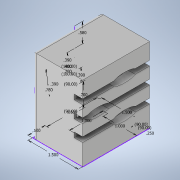
# Autodesk Inventor part: Valve Holder-3valve
Saved by Autodesk Inventor 2020 (Build 240168000, 168)
## iProperties
Created: 2022-01-25
Part Number: Valve Holder-3valve
Material: Generic
Document SubType Name: Modeling
Designer: Beaucage
Density: 1 g/cm^3
Appearance: Default
Author: Beaucage
Autodesk Inventor part; units mm, degrees
ref_plane "YZ Plane" through (0, 0, 0) normal (1, 0, 0) x (0, 1, 0)
ref_plane "XZ Plane" through (0, 0, 0) normal (0, 1, 0) x (-1, 0, 0)
ref_plane "XY Plane" through (0, 0, 0) normal (0, 0, 1) x (1, 0, 0)
sketch "Sketch1" plane through (0, 0, 0) normal (0, 1, 0) x (-1, 0, 0)
  line L0 (0, 0) -> (38.1, 0)
  line L1 (38.1, 0) -> (38.1, -38.1)
  line L2 (38.1, -38.1) -> (0, -38.1)
  line L3 (0, -38.1) -> (0, 0)
  line L4 (0, -38.1) -> (0, -31.75)
  line L5 (0, -38.1) -> (6.35, -38.1) construction
  line L6 (0, -31.75) -> (25.4, -31.75)
  line L7 (25.4, -31.75) -> (25.4, -6.35)
  line L8 (0, 0) -> (0, -38.1)
  line L9 (0, 0) -> (38.1, 0)
  line L10 (38.1, 0) -> (38.1, 12.7)
  line L11 (38.1, 12.7) -> (0, 12.7)
  line L12 (0, 12.7) -> (0, 0)
  dimension "d0" = 38.1
  dimension "d1" = 38.1
  dimension "d2" = 6.35
  dimension "d3" = 90
  dimension "d4" = 25.4
  dimension "d5" = 90
  dimension "d6" = 25.4
  dimension "d34" = 38.1
  dimension "d35" = 12.7
  constraints: 26 end point, 5 perpendicular, 4 parallel, 3 horizontal, 1 collinear
  measures "d0" distance of L1.end L2.end
  measures "d1" distance of L0.end L1.end
  measures "d2" distance of L2.end L4.end
  measures "d3" angle of L5 L4
  measures "d4" distance of L4.end L6.end
  measures "d5" angle of L4 L6
  measures "d6" distance of L6.end L7.end
  measures "d34" distance of L11.end L10.end
  measures "d35" distance of L10.end L9.end
extrude "Extrusion1" add sketch "Sketch1" along normal blind 56.896
hole "Hole1" at (-25.4, 0, -31.75) at (-25.4, 0, -6.35) direction (0, 1, 0) diameter 9.2075 depth 12.7
sketch "Sketch2" plane through (-38.1, 0, -38.1) normal (-1, 0, 0) x (0, 0, 1)
  line L0 (19.05, 0) -> (19.05, 17.78)
  line L1 (19.05, 0) -> (36.83, 0) construction
  line L2 (19.05, 17.78) -> (19.05, 27.686)
  line L3 (19.05, 17.78) -> (28.956, 17.78) construction
  line L4 (19.05, 27.686) -> (19.05, 32.766)
  line L5 (19.05, 32.766) -> (19.05, 42.672)
  circle A0 centre (19.05, 17.78) radius 9.906
  circle A1 centre (19.05, 42.672) radius 9.906
  ellipse E0 centre (19.05, 42.672) end of major axis (28.702, 42.672) minor radius 3.5267
  ellipse E1 centre (19.05, 17.78) end of major axis (28.956, 17.78) minor radius 3.6751
  line L6 (19.05, 42.672) -> (19.05, 57.404)
  line L7 (19.05, 30.226) -> (29.21, 30.226)
  line L8 (29.21, 30.226) -> (39.116, 30.226)
  circle A2 centre (39.116, 30.226) radius 9.906
  ellipse E2 centre (39.116, 30.226) end of major axis (29.21, 30.226) minor radius 3.1895
  dimension "d16" = 17.78
  dimension "d17" = 90
  dimension "d18" = 9.906
  dimension "d19" = 90
  dimension "d20" = 5.08
  dimension "d21" = 180
  dimension "d22" = 9.906
  dimension "d23" = 180
  dimension "d32" = 14.732
  dimension "d36" = 10.16
  dimension "d37" = 9.906
  dimension "d38" = 19.812
  constraints: 18 end point, 6 coincident, 5 horizontal, 3 vertical, 2 centre point, 2 collinear, 2 horizontal alignment, 2 perpendicular, 2 vertical alignment, 1 line through centre, 1 midpoint, 1 point on line, 8 other
  measures "d16" distance of L0.start L0.end
  measures "d17" angle of L1 L0
  measures "d18" distance of L0.end L2.end
  measures "d19" angle of L3 L2
  measures "d20" distance of L2.end L4.end
  measures "d21" angle of L4 L2
  measures "d22" distance of L4.end L5.end
  measures "d23" angle of L5 L4
  measures "d32" distance of L6.start L6.end
  measures "d36" distance of L7.start L7.end
  measures "d37" distance of L7.end L8.end
  measures "d38" diameter of A2
extrude "Extrusion2" cut sketch "Sketch2" against normal blind 31.75
extrude "Extrusion3" cut sketch "Sketch2" against normal blind 38.1 contours E2 | E1 L2 L0 | L0 L2 E1 | E0 L6 L5 | L5 L6 E0
sketch "Sketch3" plane through (0, 0, 0) normal (1, 0, 0) x (0, 0, -1)
  line L0 (38.1, 0) -> (38.1, 56.896) projected
  line L1 (0, 44.577) -> (38.1, 44.577)
  line L2 (38.1, 44.577) -> (38.1, 40.767)
  line L3 (38.1, 40.767) -> (0, 40.767)
  line L4 (0, 40.767) -> (0, 44.577)
  line L5 (0, 44.577) -> (38.1, 40.767) construction
  line L6 (38.1, 44.577) -> (0, 40.767) construction
  line L7 (0, 19.685) -> (38.1, 19.685)
  line L8 (38.1, 19.685) -> (38.1, 15.875)
  line L9 (38.1, 15.875) -> (0, 15.875)
  line L10 (0, 15.875) -> (0, 19.685)
  line L11 (0, 19.685) -> (38.1, 15.875) construction
  line L12 (38.1, 19.685) -> (0, 15.875) construction
  line L13 (-12.7, 0) -> (-12.7, 56.896) projected
  line L14 (0, 15.875) -> (-12.7, 15.875)
  line L15 (-12.7, 15.875) -> (-12.7, 19.685)
  line L16 (-12.7, 19.685) -> (0, 19.685)
  line L17 (0, 19.685) -> (0, 15.875)
  line L18 (0, 40.767) -> (-12.7, 40.767)
  line L19 (-12.7, 40.767) -> (-12.7, 44.577)
  line L20 (-12.7, 44.577) -> (0, 44.577)
  line L21 (0, 44.577) -> (0, 40.767)
  line L22 (-12.7, 0) -> (-12.7, 56.896) projected
  line L23 (38.1, 0) -> (38.1, 56.896) projected
  line L24 (-40.132, 28.321) -> (38.1, 28.321)
  line L25 (38.1, 28.321) -> (38.1, 32.131)
  line L26 (38.1, 32.131) -> (-40.132, 32.131)
  line L27 (-40.132, 32.131) -> (-40.132, 28.321)
  line L28 (-40.132, 28.321) -> (38.1, 32.131) construction
  line L29 (38.1, 28.321) -> (-40.132, 32.131) construction
  point P0 (0, 0)
  point P1 (19.05, 17.78)
  point P2 (19.05, 42.672)
  point P3 (-1.016, 30.226)
  point P4 (38.1, 28.321)
  dimension "d28" = 3.81
  dimension "d29" = 3.81
  dimension "d39" = 3.81
  constraints: 52 end point, 10 parallel, 6 midpoint, 5 horizontal, 5 perpendicular, 4 point on line, 2 other
  measures "d28" distance of L1.end L2.end
  measures "d29" distance of L7.end L8.end
  measures "d39" distance of L25.end L24.end
extrude "Extrusion4" cut sketch "Sketch3" against normal blind 6.35 contours L9 L10 L7 L0 | L14 L13 L16 L10 | L24 L13 L26 L0 | L24 L27 L26 L13 | L3 L4 L1 L0 | L18 L13 L20 L4
fillet "Fillet1" radius 3.175 2 edges at (-38.1, 56.896, -12.7) (-38.1, 28.448, 12.7)
body "Solid1"
